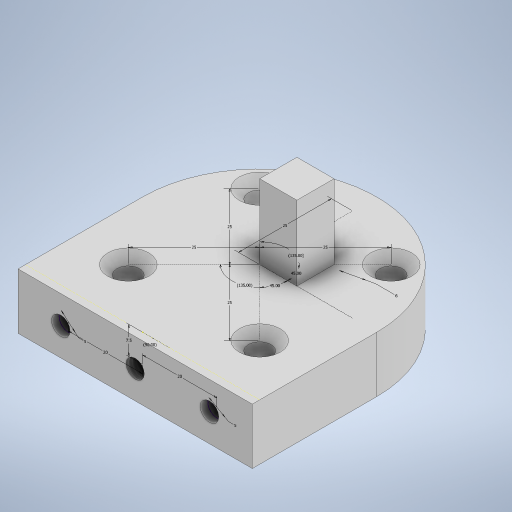
# Autodesk Inventor part: UR attachment
Saved by Autodesk Inventor 2024 (Build 280153000, 153)
## iProperties
Created: 2026-03-10
Part Number: UR attachment
Material: Generic
Document SubType Name: Modeling
Designer: Nathan
Density: 1 g/cm^3
Appearance: Default
Author: Nathan
Autodesk Inventor part; units mm, degrees
ref_plane "YZ Plane" through (0, 0, 0) normal (1, 0, 0) x (0, 1, 0)
ref_plane "XZ Plane" through (0, 0, 0) normal (0, 1, 0) x (-1, 0, 0)
sketch "Sketch1" plane through (0, 0, 0) normal (0, 1, 0) x (-1, 0, 0)
  circle A0 centre (0, 0) radius 31.5
  circle A1 centre (0, 0) radius 25
  circle A2 centre (0, 0) radius 15.75
  dimension "d0" = 63
  dimension "d1" = 50
  dimension "d2" = 31.5
  constraints: 3 centre point, 3 coincident
  measures "d0" diameter of A0
  measures "d1" diameter of A1
  measures "d2" diameter of A2
extrude "Extrusion1" add sketch "Sketch1" against normal blind 15 contours A0 | A1 | A2
sketch "Sketch2" plane through (0, 0, 0) normal (0, 1, 0) x (1, 0, 0)
  line L0 (0, 0) -> (0, 25) construction
  line L1 (0, 0) -> (17.6777, 17.6777) construction
  line L2 (0, 0) -> (25, 0) construction
  line L3 (0, 0) -> (17.6777, -17.6777) construction
  line L4 (0, 0) -> (25, 0) construction
  line L5 (0, 0) -> (-17.6777, -17.6777) construction
  line L6 (0, 0) -> (25, 0) construction
  line L7 (0, 0) -> (-17.6777, 17.6777) construction
  line L8 (0, 0) -> (25, 0) construction
  dimension "d5" = 25
  dimension "d6" = 25
  dimension "d7" = 45
  dimension "d8" = 25
  dimension "d9" = 45
  dimension "d10" = 25
  dimension "d11" = 135
  dimension "d12" = 25
  dimension "d13" = 135
  constraints: 18 end point, 4 equal length, 4 horizontal, 2 perpendicular, 1 vertical
  measures "d5" distance of L0.start L0.end
  measures "d6" distance of L0.start L1.end
  measures "d7" angle of L2 L1
  measures "d8" distance of L0.start L3.end
  measures "d9" angle of L3 L4
  measures "d10" distance of L0.start L5.end
  measures "d11" angle of L5 L6
  measures "d12" distance of L0.start L7.end
  measures "d13" angle of L8 L7
hole "Hole1" at (17.6777, 0, -17.6777) at (17.6777, 0, 17.6777) at (-17.6777, 0, 17.6777) at (-17.6777, 0, -17.6777) direction (0, -1, 0) diameter 6.1 end through all countersink diameter 11 countersink angle 90 clearance for "Countersunk Flat Head Screw ISO 2009/7046" size "M6" standard "ISO"
sketch "Sketch3" plane through (0, -15, 0) normal (0, -1, 0) x (1, 0, 0)
  circle A0 centre (17.6777, 17.6777) radius 3.05 construction
  circle A1 centre (0, 0) radius 25 construction
  circle A2 centre (0, -25) radius 3
  dimension "d39" = 6
  constraints: 2 centre point, 2 point on circle, 1 coincident
  measures "d39" diameter of A2
sketch "Sketch4" plane through (0, 0, 0) normal (0, 1, 0) x (1, 0, 0)
  line L0 (0, 0) -> (10, 0)
  line L1 (10, 0) -> (10, 10)
  line L2 (10, 10) -> (0, 10)
  line L3 (0, 10) -> (0, 0)
  dimension "d24" = 10
  dimension "d25" = 10
  constraints: 8 end point, 2 parallel, 1 horizontal, 1 perpendicular
  measures "d24" distance of L2.end L1.end
  measures "d25" distance of L1.end L0.end
extrude "Extrusion3" add sketch "Sketch4" along normal blind 20
ref_plane "Work Plane1" through (0, 0, 31.5) normal (0, 0, 1) x (1, 0, 0)
sketch "Sketch5" plane through (0, 0, 31.5) normal (0, 0, 1) x (1, 0, 0)
  line L0 (-31.5, 0) -> (-31.5, -15) projected
  line L1 (31.5, 0) -> (-31.5, 0) projected
  line L2 (31.5, -10) -> (31.5, 0)
  line L3 (31.5, 0) -> (-31.5, 0)
  line L4 (-31.5, 0) -> (-31.5, -10)
  line L5 (-31.5, -15) -> (31.5, -15) projected
  line L6 (-31.5, -10) -> (-31.5, -15)
  line L7 (-31.5, -15) -> (31.5, -15)
  line L8 (31.5, -15) -> (31.5, -10)
  point P0 (0, 0)
  constraints: 12 end point, 2 perpendicular, 1 parallel, 1 point on line, 1 vertical
extrude "Extrusion4" add sketch "Sketch5" along normal up to surface round surface about axis through (0, 0, 0) along (0, -1, 0) radius 31.5 far side no
sketch "Sketch12" plane through (0, 0, 31.5) normal (0, 0, 1) x (1, 0, 0)
  line L0 (0, 0) -> (0, -7.5) construction
  line L1 (31.5, 0) -> (-31.5, 0) construction
  line L2 (0, 0) -> (7.5, 0) construction
  dimension "d74" = 7.5
  dimension "d75" = 90
  constraints: 4 end point, 2 perpendicular, 1 horizontal
  measures "d74" distance of L0.start L0.end
  measures "d75" angle of L0 L2
sketch "Sketch13" plane through (0, 0, 31.5) normal (0, 0, 1) x (1, 0, 0)
  circle A0 centre (0, -7.5) radius 3.3 construction
  line L0 (0, -7.5) -> (20, -7.5) construction
  line L1 (0, -7.5) -> (-20, -7.5) construction
  circle A1 centre (20, -7.5) radius 2.5
  circle A2 centre (-20, -7.5) radius 2.5
  point P0 (0, 0)
  dimension "d83" = 20
  dimension "d84" = 20
  dimension "d85" = 5
  dimension "d86" = 5
  constraints: 4 end point, 2 centre point, 2 coincident, 2 horizontal
  measures "d83" distance of L0.start L0.end
  measures "d84" distance of L0.start L1.end
  measures "d85" diameter of A1
  measures "d86" diameter of A2
extrude "Extrusion13" cut sketch "Sketch3" against normal blind 6
sketch "Sketch16" plane through (0, 0, 31.5) normal (0, 0, 1) x (1, 0, 0)
  line L0 (31.5, 0) -> (-31.5, 0) projected
  line L1 (-31.5, -15) -> (31.5, -15) projected
  line L2 (-31.5, 0) -> (31.5, 0)
  line L3 (31.5, 0) -> (31.5, -15)
  line L4 (31.5, -15) -> (-31.5, -15)
  line L5 (-31.5, -15) -> (-31.5, 0)
  circle A0 centre (20, -7.5) radius 2.5 projected
  circle A1 centre (-20, -7.5) radius 2.5 projected
  line L6 (0, 0) -> (0, -7.5)
  dimension "d99" = 7.5
  constraints: 10 end point, 2 parallel, 1 horizontal, 1 perpendicular, 1 vertical
  measures "d99" distance of L6.start L6.end
extrude "Extrusion14" add sketch "Sketch16" along normal blind 2 contours L3 L1 L5 L0 | A0 | A1
sketch "Sketch17" plane through (0, 0, 33.5) normal (0, 0, 1) x (1, 0, 0)
  line L0 (0, 0) -> (0, -7.5) construction
  dimension "d102" = 7.5
  constraints: 2 end point, 1 vertical
  measures "d102" distance of L0.start L0.end
hole "Hole5" at (0, -7.5, 33.5) direction (0, 0, -1) diameter 4.917 depth 23 thread size "M6x1" class "6H" standard "ANSI Metric M Profile"
sketch "Sketch18" plane through (0, 0, 33.5) normal (0, 0, 1) x (1, 0, 0)
  line L0 (0, 0) -> (0, -7.5) construction
  line L1 (0, -7.5) -> (-20, -7.5) construction
  line L2 (0, -7.5) -> (20, -7.5) construction
  circle A0 centre (-20, -7.5) radius 2.5
  circle A1 centre (20, -7.5) radius 2.5
  dimension "d113" = 7.5
  dimension "d114" = 20
  dimension "d115" = 20
  dimension "d116" = 5
  dimension "d117" = 5
  constraints: 6 end point, 2 centre point, 2 coincident, 1 horizontal, 1 perpendicular, 1 vertical
  measures "d113" distance of L0.start L0.end
  measures "d114" distance of L0.end L1.end
  measures "d115" distance of L0.end L2.end
  measures "d116" diameter of A0
  measures "d117" diameter of A1
extrude "Extrusion15" cut sketch "Sketch18" against normal blind 11
body "Solid1"
